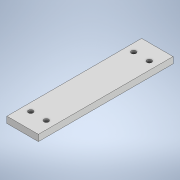
# Autodesk Inventor part: suporte estruzor 2
Saved by Autodesk Inventor 2022 (Build 260153000, 153)
## iProperties
Created: 2022-02-16
Part Number: suporte estruzor 2
Material: Genérico
Document SubType Name: Modeling
Designer: mathe
Density: 1 g/cm^3
Appearance: Padrão
Author: mathe
Autodesk Inventor part; units mm, degrees
ref_plane "YZ Plane" through (0, 0, 0) normal (1, 0, 0) x (0, 1, 0)
ref_plane "XZ Plane" through (0, 0, 0) normal (0, 1, 0) x (-1, 0, 0)
ref_plane "XY Plane" through (0, 0, 0) normal (0, 0, 1) x (1, 0, 0)
sketch "Esboço1" plane through (0, 0, 0) normal (0, 1, 0) x (-1, 0, 0)
  line L0 (0, 0) -> (19.8493, 0)
  line L1 (19.8493, 0) -> (19.8493, -85)
  line L2 (19.8493, -85) -> (0, -85)
  line L3 (0, -85) -> (0, 0)
  line L4 (20, -22) -> (20, -63)
  line L5 (0, -63) -> (0, -22)
  circle A0 centre (14.8493, -75) radius 1.5
  circle A1 centre (5, -75) radius 1.5
  circle A2 centre (14.8493, -10) radius 1.5
  circle A3 centre (5, -10) radius 1.5
  dimension "d15" = 3
  dimension "d16" = 3
  dimension "d17" = 3
  dimension "d18" = 3
  dimension "d19" = 10
  dimension "d20" = 5
  dimension "d21" = 5
  dimension "d22" = 10
  dimension "d23" = 5
  dimension "d24" = 5
  dimension "d25" = 10
  dimension "d26" = 10
  constraints: 12 end point, 4 centre point, 3 parallel, 1 horizontal, 1 perpendicular
  measures "d15" diameter of A0
  measures "d16" diameter of A1
  measures "d17" diameter of A2
  measures "d18" diameter of A3
  measures "d19" distance from line of L2 A0.centre
  measures "d20" distance from line of L1 A0.centre
  measures "d21" distance from line of L3 A1.centre
  measures "d22" distance from line of L2 A1.centre
  measures "d23" distance from line of L3 A3.centre
  measures "d24" distance from line of L1 A2.centre
  measures "d25" distance from line of L0 A3.centre
  measures "d26" distance from line of L0 A2.centre
extrude "Extrusão3" add sketch "Esboço1" along normal blind 4
